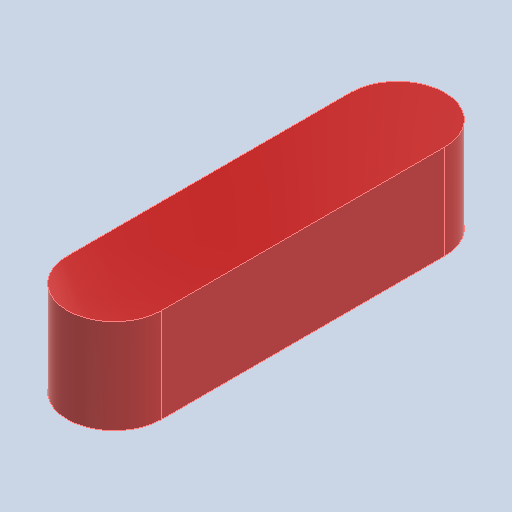
# Autodesk Inventor part: Passfeder6x3x3
Saved by Autodesk Inventor 2022 (Build 260153000, 153)
## iProperties
Created: 2022-03-11
Part Number: Passfeder6x3x3
Material: Generisch
Document SubType Name: Modeling
Designer: 123St
Density: 1 g/cm^3
Appearance: Rot
Mass: 0.138206 g
Surface Area: 1.98412 cm^2
Volume: 0.138206 cm^3
Passfeder_length: 12,000 mm
Passfeder_height: 3,000 mm
Passfeder_width: 3,000 mm
Wellennuttiefe: 1,800 mm
Nabennuttiefe: 1,400 mm
Author: 123St
Autodesk Inventor part; units mm, degrees
ref_plane "YZ Plane" through (0, 0, 0) normal (1, 0, 0) x (0, 1, 0)
ref_plane "XZ Plane" through (0, 0, 0) normal (0, 1, 0) x (-1, 0, 0)
ref_plane "XY Plane" through (0, 0, 0) normal (0, 0, 1) x (1, 0, 0)
sketch "Skizze1" plane through (0, 0, 0) normal (0, 1, 0) x (-1, 0, 0)
  line L0 (0, 4.5) -> (0, -4.5) construction
  line L1 (-1.5, 4.5) -> (-1.5, -4.5)
  line L2 (1.5, -4.5) -> (1.5, 4.5)
  arc A0 (1.5, 4.5) -> (-1.5, 4.5) centre (0, 4.5) ccw
  arc A1 (-1.5, -4.5) -> (1.5, -4.5) centre (0, -4.5) ccw
  line L3 (0, -11.2) -> (0, 11.2) construction
  point P0 (0, 0)
  point P1 (0, 0)
  point P2 (0, 6)
  point P3 (0, -6)
  dimension "d1" = 3
  dimension "d4" = 12
  constraints: 8 end point, 6 point on circle, 4 tangent, 2 centre point, 2 point on line, 1 coincident, 1 collinear, 1 midpoint, 1 parallel, 1 vertical
  measures "d1" distance between parallel lines of L1 L2
  measures "d4" distance of point (0, -6) point (0, 6)
extrude "Extrusion1" add sketch "Skizze1" along normal blind 3
equation "\"d1\" = Passfeder_width"
equation "\"d4\" = Passfeder_length"
equation "\"d2\" = Passfeder_height"
equation "\"Passfeder_height\" = 3"
equation "\"Passfeder_width\" = 3"
equation "\"Passfeder_length\" = 12"
equation "\"Wellennuttiefe\" = 1.8"
equation "\"Nabennuttiefe\" = 1.4"
